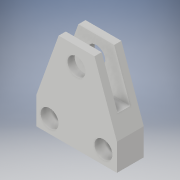
# Autodesk Inventor part: Součást9
Saved by Autodesk Inventor 2019 (Build 230136000, 136)
## iProperties
Created: 2019-11-04
Part Number: Součást9
Material: Všeobecné
Document SubType Name: Modeling
Designer: hynek
Density: 1 g/cm^3
Appearance: Výchozí
Author: hynek
Autodesk Inventor part; units mm, degrees
ref_plane "YZ Plane" through (0, 0, 0) normal (1, 0, 0) x (0, 1, 0)
ref_plane "XZ Plane" through (0, 0, 0) normal (0, 1, 0) x (-1, 0, 0)
ref_plane "XY Plane" through (0, 0, 0) normal (0, 0, 1) x (1, 0, 0)
sketch "Náčrt1" plane through (0, 0, 0) normal (0, 0, 1) x (1, 0, 0)
  line L0 (0, 0) -> (-90, 0)
  line L1 (-90, 0) -> (-90, 30)
  line L2 (-45, 0) -> (-45, 128.8279) construction
  line L3 (-45, 100) -> (-65, 100)
  line L4 (-90, 30) -> (-65, 100)
  line L5 (0, 0) -> (0, 30)
  line L6 (-45, 100) -> (-25, 100)
  line L7 (0, 30) -> (-25, 100)
  circle A0 centre (-45, 80) radius 10
  circle A1 centre (-75, 15) radius 6.5
  circle A2 centre (-75, 15) radius 10
  circle A3 centre (-15, 15) radius 6.5
  circle A4 centre (-15, 15) radius 10
  dimension "d0" = 90
  dimension "d1" = 30
  dimension "d4" = 20
  dimension "d5" = 100
  dimension "d6" = 20
  dimension "d7" = 80
  dimension "d8" = 13
  dimension "d10" = 15
  dimension "d11" = 20
  dimension "d12" = 15
  constraints: 16 end point, 5 centre point, 4 symmetric about line, 2 coincident, 2 horizontal, 2 point on line, 2 vertical, 1 midpoint, 2 other
  measures "d0" distance of L0.start L0.end
  measures "d1" distance of L0.end L1.end
  measures "d4" distance of L3.start L3.end
  measures "d5" distance between parallel lines of L0 L3
  measures "d6" diameter of A0
  measures "d7" distance from line of A0.centre L0
  measures "d8" diameter of A1
  measures "d10" distance from line of A1.centre L0
  measures "d11" diameter of A2
  measures "d12" distance from line of A1.centre L1
extrude "Vysunutí1" add sketch "Náčrt1" along normal blind 30 contours L0 L1 L4 L3 L6 L7 L5
sketch "Náčrt2" plane through (0, 0, 0) normal (0, 0, 1) x (1, 0, 0)
  circle A0 centre (-15, 15) radius 10 projected
  circle A1 centre (-75, 15) radius 10 projected
  circle A2 centre (-75, 15) radius 6.5
  circle A3 centre (-15, 15) radius 6.5
  point P0 (0, 0)
  dimension "d15" = 13
  dimension "d16" = 13
  constraints: 2 centre point, 2 coincident
  measures "d15" diameter of A3
  measures "d16" diameter of A2
extrude "Vysunutí2" add sketch "Náčrt2" along normal blind 18
sketch "Náčrt3" plane through (-90, 0, 0) normal (-1, 0, 0) x (0, 0, 1)
  line L0 (0, 30) -> (30, 30) construction
  line L1 (15, 30) -> (15, 100) construction
  line L2 (0, 100) -> (30, 100) construction
  line L3 (15, 50) -> (22, 50)
  line L4 (22, 50) -> (22, 100)
  line L5 (22, 100) -> (15, 100)
  line L6 (30, 100) -> (0, 100) construction
  line L7 (15, 50) -> (8, 50)
  line L8 (8, 50) -> (8, 100)
  line L9 (8, 100) -> (15, 100)
  point P0 (0, 0)
  dimension "d19" = 7
  dimension "d20" = 50
  constraints: 16 end point, 4 symmetric about line, 3 point on line, 2 collinear, 2 midpoint, 1 horizontal, 1 perpendicular
  measures "d19" distance of L3.start L3.end
  measures "d20" distance between parallel lines of L2 L3
extrude "Vysunutí3" cut sketch "Náčrt3" against normal through all
